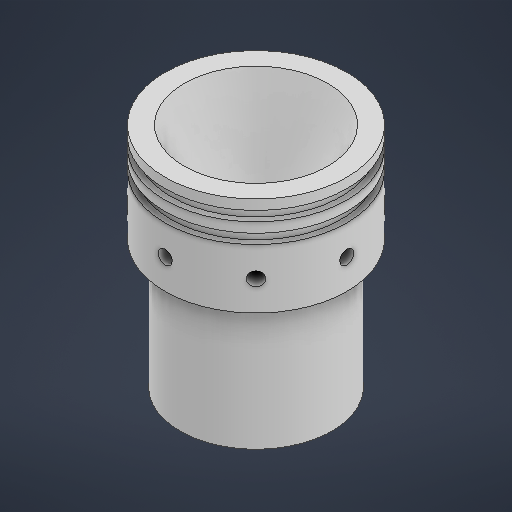
# Autodesk Inventor part: nozzle 94mm
Saved by Autodesk Inventor 2027 (Build 310192060, 192F)
## iProperties
Created: 2026-07-01
Part Number: nozzle 94mm
Material: Generic
Document SubType Name: Modeling
Designer: Alex T. Wandugu
Density: 1 g/cm^3
Appearance: Default
Matter: Mild Steel
Author: Alex T. Wandugu
Autodesk Inventor part; units mm, degrees
ref_plane "XZ Plane" through (0, 0, 0) normal (0, 1, 0) x (-1, 0, 0)
ref_plane "XY Plane" through (0, 0, 0) normal (0, 0, 1) x (1, 0, 0)
sketch "Sketch1" plane through (0, 0, 0) normal (0, 1, 0) x (-1, 0, 0)
  circle A0 centre (0, 0) radius 46
  circle A1 centre (0, 0) radius 38.445
  circle A2 centre (0, 0) radius 11.5
  dimension "d0" = 92
  dimension "d1" = 76.89
  dimension "d2" = 23
  constraints: 3 centre point, 3 coincident
  measures "d0" diameter of A0
  measures "d1" diameter of A1
  measures "d2" diameter of A2
extrude "Extrusion1" add sketch "Sketch1" against normal blind 65 contours A1
extrude "Extrusion2" add sketch "Sketch1" along normal blind 50 contours A0 | A1
sketch "Sketch2" plane through (0, 0, 0) normal (1, 0, 0) x (0, 1, 0)
  line L0 (50, -46) -> (50, 46) projected
  line L1 (0, -46) -> (0, 46) projected
  line L2 (-65, 38.445) -> (-65, -38.445) projected
  line L3 (0, -38.445) -> (0, 38.445) projected
  line L4 (0, -46) -> (0, -38.445) projected
  line L5 (0, -38.445) -> (-65, -38.445) projected
  line L6 (-65, -38.445) -> (-65, -11.5) projected
  line L7 (-65, -11.5) -> (50, -11.5) projected
  line L8 (50, -11.5) -> (50, -46) projected
  line L9 (0, 38.445) -> (0, 46) projected
  line L10 (50, 46) -> (50, 11.5) projected
  line L11 (50, 11.5) -> (-65, 11.5) projected
  line L12 (-65, 11.5) -> (-65, 38.445) projected
  line L13 (-65, 38.445) -> (0, 38.445) projected
  line L14 (45, 46) -> (40, 46)
  line L15 (40, 46) -> (40, 43)
  line L16 (40, 43) -> (45, 43)
  line L17 (45, 43) -> (45, 46)
  line L18 (35, 46) -> (30, 46)
  line L19 (30, 46) -> (30, 43)
  line L20 (30, 43) -> (35, 43)
  line L21 (35, 43) -> (35, 46)
  line L22 (-65, 11.5) -> (50, 11.5) projected
  line L23 (6, -11.5) -> (6, 11.5)
  line L24 (6, 11.5) -> (-65, 30.5244)
  line L25 (-88, 0) -> (73, 0) projected
  line L26 (-65, 30.5244) -> (-65, 0)
  line L27 (-65, 0) -> (6, 0)
  line L28 (7, 11.5) -> (7, -11.5)
  line L29 (7, 11.5) -> (50, 36.3261)
  line L30 (50, 36.3261) -> (50, 0)
  line L31 (7, 0) -> (50, 0)
  line L32 (50, -46) -> (0, -46) projected
  line L33 (0, 46) -> (50, 46) projected
  point P0 (0, 0)
  point P1 (30, 46)
  point P2 (0, 13.1077)
  point P3 (0, 0)
  dimension "d11" = 5
  dimension "d12" = 5
  dimension "d13" = 5
  dimension "d14" = 5
  dimension "d15" = 3
  dimension "d16" = 71
  dimension "d17" = 15
  dimension "d18" = 1
  dimension "d19" = 30
  constraints: 32 end point, 10 point on line, 5 parallel, 5 perpendicular, 4 midpoint, 2 horizontal
  measures "d11" distance of L14.start L0.end
  measures "d12" distance of point (40, 46) L14.start
  measures "d13" distance of L18.start point (40, 46)
  measures "d14" distance of point (30, 46) L18.start
  measures "d15" distance of L15.end L14.end
  measures "d16" distance from line of L2 L23.end
  measures "d17" angle of L25 L24
  measures "d18" distance between parallel lines of L23 L28
  measures "d19" angle of L25 L29
revolve "Revolution1" cut sketch "Sketch2" angle 360 about axis through (0, -10, 0) along (0, 1, 0) contours L25 L28 L11 L0 | L11 L29 L0 | L25 L1 L11 L23 | L25 L2 L11 L1 | L11 L1 L24 | L11 L2 L24 L1 | L17 L16 L15 L14 | L21 L20 L19 L18
ref_plane "Work Plane1" through (46, 0, 0) normal (1, 0, 0) x (0, 1, 0)
sketch "Sketch3" plane through (46, 0, 0) normal (1, 0, 0) x (0, 1, 0)
  line L0 (45, 0) -> (50, 0) projected
  line L1 (35, 0) -> (40, 0) projected
  line L2 (0, 0) -> (30, 0) projected
  circle A0 centre (15, 0) radius 3.5
  line L3 (0, -46) -> (0, 46) projected
  dimension "d23" = 7
  dimension "d24" = 15
  constraints: 1 centre point, 1 midpoint
  measures "d23" diameter of A0
  measures "d24" distance from line of L3 A0.centre
extrude "Extrusion3" cut sketch "Sketch3" against normal blind 23
pattern_circular "Circular Pattern1" count 8 over 360 about axis through (0, 0, 0) along (0, 1, 0) of "Extrusion3"
body "Solid1"
